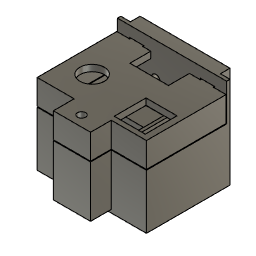
InfraredSensor (Autodesk Fusion 360 design; units mm, degrees)
Autodesk Fusion 360 part; units mm, degrees
note: some values were not read from the file. Set by a fixed rule: which sketch regions a step uses.
sketch "base" plane through (0, 0, 0) normal (0, 0, 1) x (1, 0, 0)
  line L0 (-14.605, 11.25) -> (14.605, 11.25)
  line L1 (14.605, 11.25) -> (14.605, -11.25)
  line L2 (14.605, -11.25) -> (-14.605, -11.25)
  line L3 (-14.605, -11.25) -> (-14.605, 11.25)
  line L4 (-14.605, -11.25) -> (-8.255, -11.25) construction
  line L5 (-8.255, -11.25) -> (-8.255, 2.72) construction
  line L6 (-8.255, 2.72) -> (8.255, 2.72) construction
  line L7 (-8.255, 2.72) -> (8.255, 2.72) construction
  line L8 (8.255, 2.72) -> (8.255, 0.18) construction
  line L9 (8.255, 0.18) -> (-8.255, 0.18) construction
  line L10 (-8.255, 0.18) -> (-8.255, 2.72) construction
  line L11 (-14.605, 11.25) -> (-6.405, 11.25) construction
  line L12 (-6.405, 11.25) -> (5.595, 11.25)
  line L13 (5.595, 11.25) -> (5.595, 4.75)
  line L14 (5.595, 4.75) -> (-6.405, 4.75)
  line L15 (-6.405, 4.75) -> (-6.405, 11.25)
  line L16 (14.605, -11.25) -> (5.445, -11.25)
  line L17 (5.445, -11.25) -> (5.445, -2.09)
  line L18 (5.445, -2.09) -> (14.605, -2.09)
  line L19 (14.605, -2.09) -> (14.605, -11.25)
  line L20 (8.255, 1.45) -> (-8.255, 1.45) construction
  line L21 (-2.5121, 3.45) -> (2.5121, 3.45)
  line L22 (2.5121, 3.45) -> (2.5121, -0.55)
  line L23 (2.5121, -0.55) -> (-2.5121, -0.55)
  line L24 (-2.5121, -0.55) -> (-2.5121, 3.45)
  line L25 (-0.5, 3.4446) -> (0.5, 3.4446)
  line L26 (0.5, 3.4446) -> (0.5, -0.5446)
  line L27 (0.5, -0.5446) -> (-0.5, -0.5446)
  line L28 (-0.5, -0.5446) -> (-0.5, 3.4446)
  line L29 (15.0812, 11.4622) -> (15.0812, -11.9622)
  line L30 (15.0812, -11.9622) -> (-15.0812, -11.9622)
  line L31 (-15.0812, -11.9622) -> (-15.0812, 11.4622)
  line L32 (17, -13.5) -> (-17, -13.5)
  line L33 (-17, -13.5) -> (-17, 13)
  line L34 (17, 13) -> (17, -13.5)
  line L35 (-17, 14.5) -> (17, 14.5)
  line L36 (17, 14.5) -> (17, 11.4622)
  line L37 (17, 11.4622) -> (-17, 11.4622)
  line L38 (-17, 11.4622) -> (-17, 14.5)
  line L39 (14.0812, 11.4622) -> (14.0812, -11.9622)
  line L40 (14.0812, -11.9622) -> (15.0812, -11.9622)
  line L41 (15.0812, -11.9622) -> (15.0812, 11.4622)
  line L42 (-14.0812, 11.4622) -> (-14.0812, -11.465)
  line L43 (-14.0812, -11.465) -> (-15.0812, -11.465)
  line L44 (-15.0812, -11.465) -> (-15.0812, 11.4622)
  line L45 (-15.0812, -11.9622) -> (15.0812, -11.9622)
  line L46 (15.0812, -11.9622) -> (15.0812, -10.9622)
  line L47 (15.0812, -10.9622) -> (-15.0812, -10.9622)
  line L48 (-15.0812, -10.9622) -> (-15.0812, -11.9622)
  line L49 (0.5, -11.9622) -> (-0.5, -11.9622)
  line L50 (-0.5, -11.9622) -> (-0.5, 11.4622)
  line L51 (0.5, 11.4622) -> (0.5, -11.9622)
  line L52 (-14.605, -11.25) -> (-14.605, -4.09) construction
  line L53 (-14.605, -4.09) -> (-9.305, -4.09) construction
  circle A0 centre (-9.305, -4.09) radius 3.8
  line L54 (-17, 12.5) -> (-14, 12.5)
  line L55 (-14, 12.5) -> (-14, 15.5)
  line L56 (-14, 15.5) -> (-17, 15.5)
  line L57 (-17, 15.5) -> (-17, 12.5)
  line L58 (14, 12.5) -> (17, 12.5)
  line L59 (17, 12.5) -> (17, 15.5)
  line L60 (17, 15.5) -> (14, 15.5)
  line L61 (14, 15.5) -> (14, 12.5)
  line L62 (-14, 15.5) -> (14, 15.5)
  line L63 (14.0812, -9.9755) -> (5.445, -9.9755)
  line L64 (14.0397, -2.09) -> (14.0397, -9.9755)
  point P0 (0, 1.45)
  point P1 (0, 1.45)
  dimension "d1" = 29.21
  dimension "d2" = 22.5
  dimension "d3" = 6.35
  dimension "d4" = 13.97
  dimension "d5" = 16.51
  dimension "d6" = 2.54
  dimension "d7" = 8.2
  dimension "d8" = 12
  dimension "d9" = 6.5
  dimension "d10" = 9.16
  dimension "d11" = 9.16
  dimension "d13" = 4
  dimension "d14" = 1
  dimension "d15" = 1
  dimension "d16" = 1
  dimension "d17" = 1
  dimension "d26" = 1
  dimension "d56" = 7.16
  dimension "d57" = 5.3
  dimension "d58" = 7.6
  constraint horizontal L0
  constraint perpendicular L0 L1
  constraint parallel L0 L2
  constraint parallel L1 L3
  constraint perpendicular L3 L4
  constraint perpendicular L0 L5
  constraint perpendicular L5 L6
  constraint horizontal L7
  constraint vertical L8
  constraint horizontal L9
  constraint vertical L10
  constraint perpendicular L3 L11
  constraint horizontal L12
  constraint vertical L13
  constraint horizontal L14
  constraint vertical L15
  constraint horizontal L16
  constraint vertical L17
  constraint horizontal L18
  constraint vertical L19
  constraint midpoint L8 L20.start
  constraint midpoint L10 L20.end
  constraint horizontal L21
  constraint perpendicular L21 L22
  constraint parallel L21 L23
  constraint parallel L22 L24
  constraint midpoint L20 P1
  constraint horizontal L25
  constraint perpendicular L25 L26
  constraint parallel L25 L27
  constraint parallel L26 L28
  constraint coincident P1 P0
  constraint parallel L29 L31
  constraint horizontal L32
  constraint perpendicular L32 L33
  constraint parallel L33 L34
  constraint horizontal L35
  constraint vertical L36
  constraint horizontal L37
  constraint vertical L38
  constraint coincident L34 L36.end
  constraint vertical L39
  constraint horizontal L40
  constraint vertical L41
  constraint coincident L30 L39.end
  constraint vertical L42
  constraint horizontal L43
  constraint vertical L44
  constraint horizontal L45
  constraint vertical L46
  constraint horizontal L47
  constraint vertical L48
  constraint coincident L29 L46.end
  constraint horizontal L49
  constraint perpendicular L49 L50
  constraint parallel L50 L51
  constraint coincident L30 L49.start
  constraint perpendicular L47 L52
  constraint perpendicular L42 L53
  constraint coincident L53.end A0.centre
  constraint horizontal L54
  constraint vertical L55
  constraint horizontal L56
  constraint vertical L57
  constraint coincident L38 L54.start
  constraint coincident L33 L54.start
  constraint horizontal L58
  constraint vertical L59
  constraint horizontal L60
  constraint vertical L61
  constraint perpendicular L61 L62
  constraint coincident L39 L63.start
  constraint coincident L17 L63.end
  constraint perpendicular L17 L63
  constraint coincident L18 L64.start
  constraint coincident L63 L64.end
  constraint perpendicular L63 L64
  measures "d1" distance of L1.end L2.end
  measures "d2" distance of L0.end L1.end
  measures "d3" distance of L2.end L4.end
  measures "d4" distance of L4.end L5.end
  measures "d5" distance of L5.end L6.end
  measures "d6" distance of L5.end L9.end
  measures "d7" distance of L0.start L11.end
  measures "d8" distance of L11.end L12.end
  measures "d9" distance of L11.end L14.end
  measures "d10" distance of L1.end L16.end
  measures "d11" distance of L1.end L18.end
  measures "d13" distance of L21.end L22.end
  measures "d14" distance of L26.end L27.end
  measures "d15" distance of L29.start L39.start
  measures "d16" distance of L31.end L42.start
  measures "d17" distance of L30.end L47.end
  measures "d26" distance of L50.end L51.start
  measures "d56" distance of L2.end L52.end
  measures "d57" distance of L52.end L53.end
  measures "d58" diameter of A0
extrude "Extrude1" add sketch "base" against normal blind 1.5 contours L0 L3 L31 L37 L42 L44 L47 | L0 L3 L42 L47 | L0 L12 L37 L42 L50 | L0 L14 L15 L21 L23 L24 L42 L47 L50 | L2 L3 L42 L47 | L2 L3 L31 L42 L43 L44 L47 L48 | L0 L12 L14 L15 L50 | L33 L34 L35 L36 L37 L38 L54 L55 L58 L61 | L2 L42 L47 L50 | L29 L30 L31 L32 L33 L34 L37 L40 L41 L44 L45 L46 L48 L49 | L0 L12 L37 L50 L51 | L0 L12 L14 L50 L51 | L2 L30 L31 L42 L43 L45 L48 L50 | L23 L47 L50 L51 | L2 L47 L50 L51 | L0 L12 L37 L39 L51 | L0 L12 L13 L14 L51 | L14 L21 L50 L51 | L2 L30 L45 L49 L50 L51 | L0 L13 L14 L17 L18 L21 L22 L23 L39 L47 L51 | L2 L17 L47 L51 | L0 L1 L19 L29 L37 L39 L41 L47 | L2 L16 L30 L39 L45 L51 | L2 L16 L17 L39 L47 | L17 L39 L47 L63 | L0 L1 L18 L39 | L17 L18 L63 L64 | L1 L2 L16 L19 L39 L47 | L1 L18 L19 L39 L47 | L18 L39 L63 L64 | L1 L2 L16 L19 L29 L30 L39 L40 L41 L45 L46 L47 | L35 L55 L61 L62 | A0 makes body 1
extrude "Extrude2" add sketch "base" along normal blind 12.5 contours L0 L3 L31 L37 L42 L44 L47 | L0 L3 L42 L47 | L0 L12 L37 L42 L50 | L2 L3 L42 L47 | L2 L3 L31 L42 L43 L44 L47 L48 | L2 L42 L47 L50 | L0 L12 L37 L50 L51 | L2 L30 L31 L42 L43 L45 L48 L50 | L2 L47 L50 L51 | L0 L12 L37 L39 L51 | L2 L30 L45 L49 L50 L51 | L2 L17 L47 L51 | L0 L1 L19 L29 L37 L39 L41 L47 | L2 L16 L30 L39 L45 L51 | L2 L16 L17 L39 L47 | L0 L1 L18 L39 | L1 L2 L16 L19 L39 L47 | L1 L18 L19 L39 L47 | L1 L2 L16 L19 L29 L30 L39 L40 L41 L45 L46 L47 bodies 1
extrude "Extrude3" add sketch "base" along normal blind 15.5 contours L29 L30 L31 L32 L33 L34 L37 L40 L41 L44 L45 L46 L48 L49 bodies 1
extrude "Extrude4" add sketch "base" along normal blind 27 contours L33 L34 L35 L36 L37 L38 L54 L55 L58 L61 | L35 L55 L61 L62 bodies 1
extrude "Extrude5" add sketch "base" along normal blind 10 contours L0 L12 L14 L50 L51 | L23 L47 L50 L51 | L2 L47 L50 L51 | L14 L21 L50 L51 | L23 L27 L50 L51 | L21 L25 L50 L51 | L25 L26 L27 L28 L50 L51 bodies 1
sketch "back" plane through (0, 15.5, 0) normal (0, 1, 0) x (-1, 0, 0)
  line L0 (-17, 25) -> (-17, -1.5)
  line L1 (-17, -1.5) -> (17, -1.5)
  line L2 (17, -1.5) -> (17, 25)
  line L3 (17, 25) -> (-17, 25)
  line L4 (0.0318, 16.5) -> (-4.9682, 16.5) construction
  circle A0 centre (5.0318, 16.5) radius 1.35
  line L5 (0.0318, 16.5) -> (5.0318, 16.5) construction
  circle A1 centre (-4.9682, 16.5) radius 1.35
  line L6 (0.0318, -1.5) -> (0.0318, 16.5) construction
  line L7 (-0.5, 0) -> (0.5, 0)
  line L8 (0.5, 0) -> (0.5, -1.5)
  line L9 (0.5, -1.5) -> (-0.5, -1.5)
  line L10 (-0.5, -1.5) -> (-0.5, 0)
  line L11 (-0.5, 0) -> (-0.2, -1.5)
  line L12 (0.5, 0) -> (0.2, -1.5)
  line L13 (-14.0812, 0) -> (-14.0812, 12.5)
  line L14 (14.0812, 0) -> (14.0812, 12.5)
  line L15 (17, 0) -> (-17, 0)
  line L16 (-0.5, 0) -> (-0.5, 10)
  line L17 (0.5, 10) -> (0.5, 0)
  line L18 (-0.5, 10) -> (0.5, 10)
  line L19 (-6.4216, 1.0721) -> (-1.7732, 4.8687) construction
  arc A2 (-6.4216, 1.0721) -> (-1.7732, 4.8687) centre (-4.585, 3.5673) ccw construction
  line L20 (-7.2793, 0) -> (-14.0812, 8.1062)
  line L21 (-7.2793, 0) -> (2.4108, 0) construction
  line L22 (7.3428, 0) -> (14.1447, 8.1062)
  line L23 (-14.0812, 8.1062) -> (14.1447, 8.1062)
  line L24 (-14, 27) -> (-14, -1.5)
  line L25 (-14, -1.5) -> (14, -1.5)
  line L26 (14, -1.5) -> (14, 27)
  line L27 (14, 27) -> (-14, 27)
  dimension "d29" = 18
  dimension "d30" = 5
  dimension "d31" = 5
  dimension "d32" = 2.7
  dimension "d33" = 2.7
  dimension "d42" = 1
  dimension "d47" = 130
  constraint perpendicular L4 L6
  constraint perpendicular L5 L6
  constraint coincident L4.end A1.centre
  constraint coincident A0.centre L5.end
  constraint horizontal L7
  constraint vertical L8
  constraint horizontal L9
  constraint vertical L10
  constraint coincident L1 L8.end
  constraint coincident L9 L11.end
  constraint coincident L9 L12.end
  constraint horizontal L21
  constraint coincident L15 L20.start
  constraint coincident L13 L20.end
  constraint symmetric L6 L20.start L22.start
  constraint symmetric L6 L20.end L22.end
  constraint perpendicular L14 L23
  measures "d29" distance of L4.start L6.start
  measures "d30" distance of L4.start L4.end
  measures "d31" distance of L4.start A0.centre
  measures "d32" diameter of A1
  measures "d33" diameter of A0
  measures "d42" distance of L7.start L7.end
  measures "d47" angle of L20 L21
extrude "Extrude6" cut sketch "back" against normal blind 6 contours A0 | A1 bodies 1
extrude "Extrude9" add sketch "back" along normal blind -3 and the other way blind 26.4622 contours L13 L15 L20 L24 | L15 L20 L24 | L15 L22 L26 | L14 L15 L22 L26 bodies 1
extrude "Extrude10" add sketch "back" along normal blind -19 and the other way blind 27 separate body contours L20 L23 L24 | L15 L16 L20 L23 L24 | L15 L17 L22 L23 L26 | L14 L22 L23 L26 | L14 L22 L23 makes body 2 at (-5.0482, -8.8333, 8.1062) makes body 3 at (9.5541, -8.8333, 8.1062)
copy_body "CopyPasteBodies1" bodies 3 2 makes body 4 makes body 5
move_body "Move1" bodies 4 5 to x (1, 0, 0) y (0, 1, 0) z (0, 0, 1) at (0, 16.5, 0)
extrude "Extrude16" cut 1 faces at (-7.3292, 13, 5.4042) along direction (0, -1, 0) blind 0.5 on bodies 5 bodies 5
combine "Combine1" operation add target body 1 tool bodies 2 3 4 5
sketch "top" plane through (0, 0, 15.5) normal (0, 0, 1) x (-1, 0, 0)
  line L0 (15.0812, -11.4622) -> (17, -11.4622)
  line L1 (17, -11.4622) -> (17, 13.5)
  line L2 (17, 13.5) -> (-17, 13.5)
  line L3 (-17, 13.5) -> (-17, -11.4622)
  line L4 (-17, -11.4622) -> (-15.0812, -11.4622)
  line L5 (-15.0812, -11.4622) -> (-15.0812, 11.9622)
  line L6 (-15.0812, 11.9622) -> (15.0812, 11.9622)
  line L7 (15.0812, 11.9622) -> (15.0812, -11.4622)
  line L8 (-17, -13) -> (-17, 13.5)
  line L9 (-15.0812, -11.4622) -> (-15.0812, 11.9622)
  line L10 (-17, -11.4622) -> (17, -11.4622)
  line L11 (15.0812, 11.465) -> (15.0812, -11.4622)
  line L12 (17, 13.5) -> (17, -13)
  line L13 (-17, 13.5) -> (17, 13.5)
  line L14 (-5.595, -11.25) -> (-5.595, -4.75)
  line L15 (-5.595, -4.75) -> (6.405, -4.75)
  line L16 (6.405, -4.75) -> (6.405, -11.25)
  line L17 (-5.445, 11.25) -> (-5.445, 2.09)
  line L18 (-5.445, 2.09) -> (-14.605, 2.09)
  circle A0 centre (9.305, 4.09) radius 3.8
  line L19 (-14.605, 2.09) -> (-15.0812, 2.09)
  line L20 (-5.445, 11.25) -> (-5.445, 11.9622)
  line L21 (-5.595, -11.25) -> (-5.595, -11.4622)
  line L22 (6.405, -11.25) -> (6.405, -11.4622)
  line L23 (12.9907, -11.4622) -> (8.9907, -11.4622)
  line L24 (8.9907, -11.4622) -> (8.9907, -12.9622)
  line L25 (8.9907, -12.9622) -> (12.9907, -12.9622)
  line L26 (12.9907, -12.9622) -> (12.9907, -11.4622)
  line L27 (-9.0093, -11.4622) -> (-13.0093, -11.4622)
  line L28 (-13.0093, -11.4622) -> (-13.0093, -12.9622)
  line L29 (-13.0093, -12.9622) -> (-9.0093, -12.9622)
  line L30 (-9.0093, -12.9622) -> (-9.0093, -11.4622)
  line L31 (2.722, 11.9622) -> (-2, 11.9622)
  line L32 (-2, 11.9622) -> (-2, 10)
  line L33 (-2, 10) -> (2.722, 10)
  line L34 (2.722, 10) -> (2.722, 11.9622)
  circle A1 centre (0, 16.7) radius 0.9
  circle A2 centre (0, 16.7) radius 1.25
  line L35 (5.4974, 13.5) -> (-6.0721, 13.5)
  line L36 (-6.0721, 13.5) -> (-6.0721, 19.9617)
  line L37 (-6.0721, 19.9617) -> (5.4974, 19.9617)
  line L38 (5.4974, 19.9617) -> (5.4974, 13.5)
  line L39 (-14.0812, 9.9755) -> (-5.445, 9.9755)
  line L40 (-14.0397, 2.09) -> (-14.0397, 9.9755)
  dimension "d65" = 4
  dimension "d66" = 1.5
  dimension "d67" = 4
  dimension "d68" = 1.5
  dimension "d76" = 1.8
  dimension "d77" = 2.5
  constraint coincident L18.end L19.start
  constraint coincident L9 L19.end
  constraint perpendicular L9 L19
  constraint coincident L17.start L20.start
  constraint coincident L6 L20.end
  constraint perpendicular L6 L20
  constraint coincident L14.start L21.start
  constraint coincident L10 L21.end
  constraint perpendicular L10 L21
  constraint coincident L16.end L22.start
  constraint coincident L10 L22.end
  constraint perpendicular L10 L22
  constraint horizontal L23
  constraint vertical L24
  constraint horizontal L25
  constraint vertical L26
  constraint coincident L10 L23.start
  constraint horizontal L27
  constraint vertical L28
  constraint horizontal L29
  constraint vertical L30
  constraint horizontal L31
  constraint vertical L32
  constraint horizontal L33
  constraint vertical L34
  constraint coincident L6 L31.start
  constraint concentric A1 A2
  constraint horizontal L35
  constraint vertical L36
  constraint horizontal L37
  constraint vertical L38
  constraint coincident L2 L35.start
  measures "d65" distance of L23.start L23.end
  measures "d66" distance of L23.start L25.end
  measures "d67" distance of L27.start L27.end
  measures "d68" distance of L27.start L29.end
  measures "d76" diameter of A1
  measures "d77" diameter of A2
extrude "Extrude11" add sketch "top" along normal blind 6 separate body contours L0 L1 L2 L3 L4 L5 L6 L7 L8 L9 L10 L11 L12 L13 L31 L35 makes body 6
extrude "Extrude12" add sketch "top" along normal blind 8 and the other way blind -6 separate body contours L0 L1 L2 L3 L4 L5 L6 L7 L8 L9 L10 L11 L12 L13 L31 L35 | L5 L6 L7 L9 L10 L11 L14 L15 L16 L17 L18 L19 L20 L21 L22 L23 L27 L32 L33 L34 | L10 L23 L24 L25 L26 | L6 L31 L32 L33 L34 | L10 L27 L28 L29 L30 makes body 7
extrude "Extrude13" add sketch "top" along normal blind 7 and the other way blind 1.2 contours L6 L31 L32 L33 L34 bodies 7 6
combine "Combine2" operation cut target body 1 tool bodies 7 keep tools
move_face "OffsetFaces1" offset -0.2 9 faces at (-8.9907, 11.9622, 22.8333) (-10.3241, 11.9622, 23.5) (-11.6574, 12.4622, 21.5) (-12.9907, 12.4622, 22.8333) (9.0093, 12.4622, 22.8333) (10.3426, 12.4622, 21.5) (10.3426, 12.4622, 23.5) (13.0093, 11.9622, 22.8333) (-10.3241, 12.9622, 22.1667) on bodies 1
move_face "OffsetFaces2" offset -0.2 5 faces at (16.3604, 11.4622, 20.1667) (7.8712, 11.4622, 22.1667) (-7.2669, 11.4622, 22.1667) (-16.3604, 11.4622, 20.1667) (-16.3604, -4.6667, 15.5) on bodies 7
move_face "OffsetFaces3" offset -0.2 1 faces at (0.426, -11.9622, 14.7667) on bodies 7
extrude "Extrude14" add sketch "top" along normal blind 8 contours L2 L13 L35 L36 L37 L38 bodies 7
move_face "OffsetFaces4" offset -0.2 1 faces at (4.4647, -16.7206, 15.5) on bodies 7
extrude "Extrude15" add sketch "top" against normal blind 16 contours L2 L13 L35 L36 L37 L38 | A2 bodies 1
named bodies: "sensor_housing2", "sensor top2", "sensor_top2"
